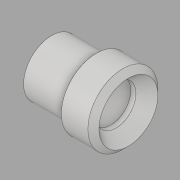
# Autodesk Inventor part: AN929-8D
Saved by Autodesk Inventor 2019 (Build 230136000, 136)
## iProperties
Created: 2018-11-23
Part Number: AN929-8D
Material: Aluminum 2014-T6
Document SubType Name: Modeling
Designer: erics
Mass: 8.27816 g
Surface Area: 14.5162 cm^2
Volume: 2.96786 cm^3
Density: 2.78927 g/cm^3
Appearance: Satin
Author: erics
Autodesk Inventor part; units mm, degrees
ref_plane "YZ Plane" through (0, 0, 0) normal (1, 0, 0) x (0, 1, 0)
ref_plane "XZ Plane" through (0, 0, 0) normal (0, 1, 0) x (-1, 0, 0)
ref_plane "XY Plane" through (0, 0, 0) normal (0, 0, 1) x (1, 0, 0)
sketch "Sketch1" plane through (0, 0, 0) normal (0, 0, 1) x (1, 0, 0)
  line L0 (0, 0) -> (0, 6.9469)
  line L1 (0, 6.9469) -> (10.8458, 6.9469)
  line L2 (11.0998, 7.2009) -> (11.0998, 8.6741)
  line L3 (11.0998, 8.6741) -> (17.6784, 8.6741)
  line L4 (19.05, 8.6741) -> (19.05, 7.3025) construction
  line L5 (19.05, 7.3025) -> (15.949, 4.9657)
  line L6 (15.949, 4.9657) -> (14.6812, 4.9657)
  line L7 (0, 0) -> (11.6975, 0)
  line L8 (11.6975, 0) -> (14.6812, 4.9657)
  line L9 (19.05, 7.3025) -> (17.6784, 8.6741)
  line L10 (17.6784, 8.6741) -> (19.05, 8.6741) construction
  arc A0 (10.8458, 6.9469) -> (11.0998, 7.2009) centre (10.8458, 7.2009) ccw
  point P0 (11.0998, 6.9469)
  dimension "d0" = 6.9469
  dimension "d1" = 8.6741
  dimension "d2" = 7.9502
  dimension "d3" = 19.05
  dimension "d4" = 4.9657
  dimension "d5" = 4.3688
  dimension "d6" = 37
  dimension "d7" = 7.3025
  dimension "d8" = 59
  dimension "d9" = 45
  dimension "d11" = 0.254
  constraints: 22 end point, 6 perpendicular, 2 point on circle, 2 point on line, 2 tangent, 1 centre point, 1 horizontal, 1 parallel, 1 vertical
  measures "d0" distance of L0.start L0.end
  measures "d1" distance from line of L0.start L3
  measures "d2" distance between parallel lines of L4 L2
  measures "d3" distance between parallel lines of L0 L4
  measures "d4" distance from line of L0.start L6
  measures "d5" distance from line of L4 L6.end
  measures "d6" angle of L3 L5
  measures "d7" vertical distance of L4.end L0.start
  measures "d8" angle of L7 L8
  measures "d9" angle of L3 L9
  measures "d11" radius of A0
revolve "Revolution1" add sketch "Sketch1" angle 360 about axis through (0, 0, 0) along (1, 0, 0)
equation "\"d0\" = 0.5 * AN929_C"
equation "\"d1\" = 0.5 * AN929_B"
equation "\"d2\" = AN929_D"
equation "\"d3\" = AN929_H"
equation "\"d4\" = 0.5 * AN929_F"
equation "\"d5\" = AN929_E"
equation "\"d7\" = 0.5 * AN929_G"
equation "\"d11\" = AN929_R"
equation "\"Tube_OD\" = 12.7"
equation "\"AN929_B\" = 17.3482"
equation "\"AN929_C\" = 13.8938"
equation "\"AN929_D\" = 7.9502"
equation "\"AN929_E\" = 4.3688"
equation "\"AN929_F\" = 9.9314"
equation "\"AN929_G\" = 14.605"
equation "\"AN929_H\" = 19.05"
equation "\"AN929_R\" = 0.254"
body "Solid1"
